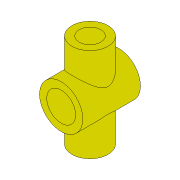
# Autodesk Inventor part: Crank
Saved by Autodesk Inventor 2022.5 (Build 265521000, 521)
## iProperties
Created: 2018-04-07
Part Number: Crank
Document SubType Name: Modeling
Designer: Administrator
Density: 1 g/cm^3
Mass: 13.3542 g
Surface Area: 74.9872 cm^2
Volume: 13.3542 cm^3
Material: Generic
Appearance: Clear - Yellow
Author: Administrator
Autodesk Inventor part; units mm, degrees
ref_plane "YZ Plane" through (0, 0, 0) normal (1, 0, 0) x (0, 1, 0)
ref_plane "XZ Plane" through (0, 0, 0) normal (0, 1, 0) x (-1, 0, 0)
ref_plane "XY Plane" through (0, 0, 0) normal (0, 0, 1) x (1, 0, 0)
sketch "Sketch8" plane through (0, 0, 0) normal (1, 0, 0) x (0, 1, 0)
  line L0 (0, 0) -> (0, -26)
  line L1 (0, -26) -> (10, -26)
  line L2 (0, 0) -> (16, 0) construction
  line L3 (10, -26) -> (10, 0)
  line L4 (0, 0) -> (0, 26)
  line L5 (0, 26) -> (10, 26)
  line L6 (10, 26) -> (10, 0)
  line L7 (6, -26) -> (6, 26)
  dimension "d26" = 26
  dimension "d27" = 16
  dimension "d28" = 10
  dimension "d29" = 6
  constraints: 16 end point, 3 perpendicular, 3 point on line, 2 symmetric about line, 1 horizontal, 1 vertical
  measures "d26" distance of L0.start L0.end
  measures "d27" distance of L0.start L2.end
  measures "d28" distance of L0.end L1.end
  measures "d29" distance between parallel lines of L7 L0
revolve "Revolution1" add sketch "Sketch8" angle 360 about axis through (0, 0, 0) along (0, 0, 1) contours L7 L5 L6 L3 L1
sketch "Sketch9" plane through (0, 0, 0) normal (1, 0, 0) x (0, 1, 0)
  line L0 (0, 0) -> (16, 0)
  line L1 (16, 0) -> (16, 12)
  line L2 (16, 12) -> (0, 12)
  line L3 (0, 12) -> (0, 0)
  line L4 (0, 0) -> (-16, 0)
  line L5 (-16, 0) -> (-16, 12)
  line L6 (-16, 12) -> (0, 12)
  line L7 (0, 12) -> (0, 0)
  dimension "d31" = 16
  dimension "d32" = 16
  dimension "d33" = 12
  constraints: 16 end point, 5 parallel, 2 horizontal, 2 perpendicular
  measures "d31" distance of L1.end L2.end
  measures "d32" distance between parallel lines of L5 L3
  measures "d33" distance of L0.end L1.end
revolve "Revolution2" add sketch "Sketch9" angle 360 about axis through (0, 0, 0) along (0, 1, 0)
sketch "Sketch10" plane through (0, 16, 0) normal (0, 1, 0) x (1, 0, 0)
  circle A0 centre (0, 0) radius 8
  dimension "d35" = 16
  constraints: 1 centre point, 1 coincident
  measures "d35" diameter of A0
extrude "Extrusion8" cut sketch "Sketch10" against normal through all
sketch "Sketch11" plane through (0, 0, 26) normal (0, 0, 1) x (1, 0, 0)
  circle A0 centre (0, 0) radius 6 projected
extrude "Extrusion9" cut sketch "Sketch11" against normal through all
body "Solid2"
